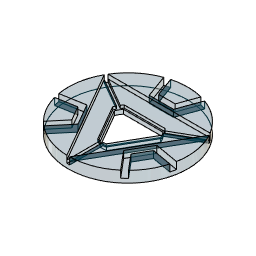
亚克力1 v18 v2 (Autodesk Fusion 360 design; units mm, degrees)
Autodesk Fusion 360 part; units mm, degrees
sketch "草图1" plane through (0, 0, 0) normal (0, 0, 1) x (1, 0, 0)
  line L0 (14.7309, 12) -> (-14.7309, 12)
  line L1 (37.729, 20.6282) -> (1, -42.9884)
  arc A0 (17.7578, 6.7574) -> (14.7309, 12) centre (0, 0) ccw
  line L2 (5.9345, 28) -> (10.9481, 41.7749)
  line L3 (15.9317, 10.3529) -> (36.729, 22.3602)
  line L4 (8.7353, 24) -> (14.7069, 40.4068)
  arc A1 (-14.7309, 12) -> (-17.7578, 6.7574) centre (0, 0) ccw
  arc A2 (-3.0268, -18.7574) -> (3.0268, -18.7574) centre (0, 0) ccw
  line L5 (0, 0) -> (-41.5692, 24) construction
  line L6 (21.2815, -19.1394) -> (27.2159, -8.8606)
  line L7 (3.0268, -18.7574) -> (17.7578, 6.7574)
  arc A3 (-14.2478, 11) -> (-16.6502, 6.839) centre (0, 0) ccw
  line L8 (-25.1523, -4.435) -> (-42.3467, -7.4669)
  line L9 (-15.9317, 10.3529) -> (-36.729, 22.3602)
  line L10 (-16.417, -19.565) -> (-27.6399, -32.9399)
  line L11 (-16.9317, 8.6208) -> (-37.729, 20.6282)
  line L12 (16.417, -19.565) -> (27.6399, -32.9399)
  line L13 (14.2478, 11) -> (-14.2478, 11)
  circle A4 centre (0, 0) radius 43
  arc A5 (16.6502, 6.839) -> (14.2478, 11) centre (0, 0) ccw
  line L14 (2.4024, -17.839) -> (16.6502, 6.839)
  line L15 (21.2815, -19.1394) -> (30.704, -30.3688)
  line L16 (-36.729, 22.3602) -> (36.729, 22.3602)
  line L17 (-17.7578, 6.7574) -> (-3.0268, -18.7574)
  line L18 (16.9317, 8.6208) -> (37.729, 20.6282)
  line L19 (27.2159, -8.8606) -> (41.6521, -11.4061)
  line L20 (25.1523, -4.435) -> (42.3467, -7.4669)
  arc A6 (-2.4024, -17.839) -> (2.4024, -17.839) centre (0, 0) ccw
  line L21 (-16.6502, 6.839) -> (-2.4024, -17.839)
  line L22 (16.417, -19.565) -> (25.1523, -4.435)
  line L23 (-1, -18.9737) -> (-1, -42.9884)
  line L24 (-8.7353, 24) -> (-14.7069, 40.4068)
  line L25 (8.0351, 25) -> (-8.0351, 25)
  line L26 (-5.9345, 28) -> (-10.9481, 41.7749)
  line L27 (-25.1523, -4.435) -> (-16.417, -19.565)
  line L28 (-21.2815, -19.1394) -> (-30.704, -30.3688)
  line L29 (0, 0) -> (0, -48) construction
  line L30 (5.9345, 28) -> (-5.9345, 28)
  line L31 (1, -18.9737) -> (1, -42.9884)
  line L32 (8.7353, 24) -> (-8.7353, 24)
  line L33 (-27.2159, -8.8606) -> (-41.6521, -11.4061)
  line L34 (-27.2159, -8.8606) -> (-21.2815, -19.1394)
  line L35 (-37.729, 20.6282) -> (-1, -42.9884)
  dimension "d1" = 4
  dimension "d6" = 360
  dimension "d7" = 1
  dimension "d8" = 120
  dimension "d9" = 1
  constraint coincident A0.centre A1.centre
  constraint coincident A0.start A1
  constraint coincident A2.start A1
  constraint coincident A2.end A1
  constraint concentric A1 A2
  constraint concentric A0 A2
  constraint vertical L29
  constraint coincident L10.end A4
  constraint coincident L23.start A2
  constraint coincident L23.end A4
  constraint parallel L23 L29
  constraint coincident L31.start A2
  constraint coincident L1.end A4
  constraint parallel L23 L31
  constraint parallel L1 L6
  constraint horizontal L16
  measures "d8" angle of L5 L29
  measures "d9" distance of L29 L31
extrude "拉伸1" add sketch "草图1" against normal blind 3 contours L0 A0 A1 A2 L7 L17 | L0 A0 L3 A1 L9 L16 | A0 L3 A4 L18 | A1 L9 L11 A4 | L1 A0 A2 L7 L18 L31 | L4 A4 L16 L24 L32 | A1 A2 L11 L17 L23 L35 | L1 L12 A4 L20 L22 | L2 L4 A4 L24 L26 L30 L32 | L8 L10 A4 L27 L35 | A2 A4 L23 L31 | L2 A4 L26 L30 | L8 L10 A4 L27 L28 L33 L34 | L6 L12 A4 L15 L19 L20 L22 | A4 L28 L33 L34 | L6 A4 L15 L19 | A3 L13 A5 L14 A6 L21 makes body 1
extrude "拉伸2" add sketch "草图1" along normal blind 5 contours L4 A4 L16 L24 L32 | L1 L12 A4 L20 L22 | L8 L10 A4 L27 L35 | L2 A4 L26 L30 | A4 L28 L33 L34 | L6 A4 L15 L19 bodies 1
extrude "拉伸3" add sketch "草图1" along normal blind 2 contours L0 A0 L3 A1 L9 L16 | L1 A0 A2 L7 L18 L31 | A1 A2 L11 L17 L23 L35 bodies 1
extrude "拉伸4" cut sketch "草图1" against normal blind 7 contours A3 L13 A5 L14 A6 L21 bodies 1
copy_body "实体->零部件2" bodies 1 removing the originals makes body 2 in component "亚克力1"
component "亚克力1" placed x (1, 0, 0) y (0, 1, 0) z (0, 0, 1) at (0, 0, 0)
